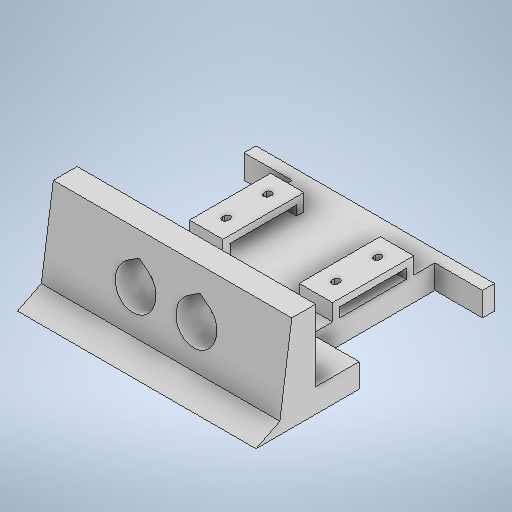
# Autodesk Inventor part: shell_01
Saved by Autodesk Inventor 2025.2 (Build 292293000, 293)
## iProperties
Created: 2025-11-21
Part Number: shell_01
Material: Generic
Document SubType Name: Modeling
Designer: Leo
Density: 1 g/cm^3
Appearance: Default
Author: Leo
Autodesk Inventor part; units mm, degrees
ref_plane "YZ Plane" through (0, 0, 0) normal (1, 0, 0) x (0, 1, 0)
ref_plane "XZ Plane" through (0, 0, 0) normal (0, 1, 0) x (-1, 0, 0)
ref_plane "XY Plane" through (0, 0, 0) normal (0, 0, 1) x (1, 0, 0)
sketch "Sketch3" plane through (0, 0, 0) normal (0, 1, 0) x (-1, 0, 0)
  line L0 (50, 50) -> (-50, 50)
  line L1 (-50, 50) -> (-50, -50)
  line L2 (-50, -50) -> (50, -50)
  line L3 (50, -50) -> (50, 50)
  line L4 (50, 50) -> (-50, -50) construction
  line L5 (-50, 50) -> (50, -50) construction
  line L6 (45, -45) -> (-45, 45) construction
  line L7 (-45, -45) -> (45, 45) construction
  point P0 (0, 0)
  dimension "d12" = 100
  dimension "d13" = 100
  constraints: 16 end point, 4 midpoint, 2 parallel, 1 horizontal, 1 perpendicular
  measures "d12" distance of L2.end L1.end
  measures "d13" distance of L0.end L1.end
extrude "Solid Mass" add sketch "Sketch3" along normal blind 40
sketch "Sketch6" plane through (50, 0, 50) normal (1, 0, 0) x (0, 0, -1)
  line L0 (0, 0) -> (100, 0) projected
  line L1 (0, 0) -> (10, 5)
  line L2 (10, 5) -> (15, 40)
  line L3 (0, 40) -> (100, 40) projected
  line L4 (0, 0) -> (0, 40)
  line L5 (100, 40) -> (25, 40)
  line L6 (25, 40) -> (25, 10)
  line L7 (25, 10) -> (100, 10)
  line L8 (100, 10) -> (100, 40)
  circle A0 centre (69.125, 22) radius 22.5
  line L9 (63.125, 17) -> (75.125, 17)
  line L10 (75.125, 17) -> (75.125, 27)
  line L11 (75.125, 27) -> (63.125, 27)
  line L12 (63.125, 27) -> (63.125, 17)
  line L13 (63.125, 17) -> (75.125, 27) construction
  line L14 (75.125, 17) -> (63.125, 27) construction
  line L15 (100, 0) -> (100, 40) projected
  line L16 (52.125, 10) -> (52.125, 17)
  line L17 (55.125, 10) -> (55.125, 14)
  line L18 (55.125, 14) -> (63.125, 14)
  line L19 (63.125, 14) -> (63.125, 10)
  line L20 (69.125, 22) -> (69.125, 0)
  line L21 (52.125, 17) -> (69.125, 17)
  line L22 (86.125, 10) -> (86.125, 17)
  line L23 (83.125, 10) -> (83.125, 14)
  line L24 (83.125, 14) -> (75.125, 14)
  line L25 (75.125, 14) -> (75.125, 10)
  line L26 (86.125, 17) -> (69.125, 17)
  point P0 (50, 0)
  point P1 (25, 40)
  point P2 (82.625, 40)
  point P3 (88.1579, 10)
  point P4 (64.408, 0)
  point P5 (50.0921, 10)
  point P6 (67.25, 14)
  point P7 (55.625, 40)
  point P8 (55.25, 14)
  point P9 (73.842, 0)
  point P10 (75.125, 10)
  point P11 (83.125, 10)
  point P12 (86.125, 10)
  point P13 (75.125, 17)
  dimension "d20" = 10
  dimension "d21" = 5
  dimension "d22" = 15
  dimension "d25" = 10
  dimension "d27" = 45
  dimension "d28" = 12
  dimension "d29" = 10
  dimension "d35" = 15
  dimension "d45" = 22
  dimension "d47" = 30.875
  dimension "d48" = 3
  dimension "d49" = 3
  dimension "d50" = 11
  constraints: 48 end point, 7 point on line, 6 symmetric about line, 5 perpendicular, 4 parallel, 4 vertical, 2 horizontal, 2 midpoint, 1 centre point, 1 collinear
  measures "d20" horizontal distance of L0.start L1.end
  measures "d21" vertical distance of L0.start L1.end
  measures "d22" horizontal distance of L0.start L2.end
  measures "d25" distance between parallel lines of L7 L0
  measures "d27" diameter of A0
  measures "d28" distance of L11.end L10.end
  measures "d29" distance of L10.end L9.end
  measures "d35" horizontal distance of L6.end L1.end
  measures "d45" distance from line of L0 L20.start
  measures "d47" distance of L0.end L20.end
  measures "d48" distance between parallel lines of L17 L16
  measures "d49" distance between parallel lines of L21 L18
  measures "d50" distance between parallel lines of L16 L19
extrude "Cut Ramp" cut sketch "Sketch6" against normal through all contours L4 L3 L2 L1 | A0 L3 L7 L22 L26 L10 L11 L12 L21 L16 | L7 L6 L3 A0 | L20 L9 L26 L22 L7 L23 L24 L25 | L7 L19 L18 L17 L16 L21 L9 L20 | A0 L3 L8 L7 | L7 L17 L18 L19 | L25 L24 L23 L7 | L9 L12 L11 L10
sketch "Sketch7" plane through (50, 10, 25) normal (0, 0, -1) x (-1, 0, 0)
  circle A0 centre (62.75, 11) radius 8.5
  line L0 (100, 0) -> (0, 0) projected
  line L1 (0, 30) -> (100, 30) projected
  line L2 (0, 0) -> (0, 30) projected
  line L3 (0, -10) -> (0, 0) projected
  line L4 (100, -10) -> (100, 0) projected
  line L5 (100, 30) -> (100, 0) projected
  line L6 (0, -10) -> (100, -10) projected
  line L7 (50, 30) -> (50, 0)
  circle A1 centre (37.25, 11) radius 8.5
  line L8 (58.2723, 18.225) -> (62.75, 21)
  line L9 (62.75, 21) -> (67.2277, 18.225)
  line L10 (41.7277, 18.225) -> (37.25, 21)
  line L11 (37.25, 21) -> (32.7723, 18.225)
  point P0 (50, -10)
  point P1 (32.7723, 18.225)
  point P2 (41.7277, 18.225)
  dimension "d30" = 17
  dimension "d31" = 11
  dimension "d32" = 25.5
  dimension "d46" = 10
  constraints: 10 end point, 4 symmetric about line, 2 centre point, 2 midpoint, 2 point on circle, 2 tangent, 1 vertical alignment, 1 other
  measures "d30" diameter of A0
  measures "d31" distance from line of L0 A0.centre
  measures "d32" diameter of A0.centre L7
  measures "d46" distance of A0.centre L8.end
extrude "Eyes" cut sketch "Sketch7" against normal through all contours A0 | A0 L8 L9 | A1 | A1 L11 L10
extrude "Motor Platform" add sketch "Sketch6" against normal up to surface (100 mm away) contours L20 L9 L26 L22 L7 L23 L24 L25 | L7 L19 L18 L17 L16 L21 L9 L20
sketch "Sketch9" plane through (-50, 0, -50) normal (-1, 0, 0) x (0, 0, 1)
  line L0 (5, 22) -> (5, 0)
  line L1 (56.75, 22) -> (56.75, 0)
  arc A0 (56.75, 22) -> (5, 22) centre (30.875, 22) ccw
  line L2 (5, 0) -> (56.75, 0)
  line L3 (0, 10) -> (13.875, 10) projected
  line L4 (24.875, 17) -> (24.875, 27) projected
  line L5 (24.875, 27) -> (36.875, 27) projected
  line L6 (36.875, 27) -> (36.875, 17) projected
  line L7 (13.875, 17) -> (47.875, 17) projected
  line L8 (13.875, 10) -> (0, 10) projected
  circle A1 centre (30.875, 22) radius 22.5 projected
  line L9 (0, 0) -> (100, 0) projected
  line L10 (0, 0) -> (0, 10) projected
  point P0 (50, 0)
  point P1 (5, 10)
  point P2 (26.158, 0)
  point P3 (11.8421, 10)
  point P4 (35.592, 0)
  dimension "d54" = 5
  dimension "d55" = 51.75
  dimension "d56" = 22
  constraints: 6 end point, 2 horizontal alignment, 2 point on circle, 1 centre point, 1 parallel, 1 point on line, 1 tangent, 1 vertical
  measures "d54" distance of L0.end L9.start
  measures "d55" distance of L0.start L1.start
  measures "d56" distance of L0.start L0.end
extrude "Cut right wheel" cut sketch "Sketch9" against normal blind 20 contours A0 L1 L2 A1 L3 L0 | L3 A1 L2 L0 | A1 L2 | L4 L5 L6 L7 picked at (31.5427, 32.8036)
extrude "Cut left wheel" cut sketch "Sketch9" along normal blind 20 from surface at -100 contours A0 L1 L2 A1 L3 L0 | L3 A1 L2 L0 | A1 L2 | L4 L5 L6 L7 picked at (31.5427, 32.8036)
sketch "Sketch8" plane through (50, 10, 25) normal (0, 1, 0) x (1, 0, 0)
  line L0 (-27, 35) -> (-27, 36) construction
  line L1 (-25.75, 35) -> (-25.75, 36)
  line L2 (-28.25, 36) -> (-28.25, 35)
  arc A0 (-28.25, 35) -> (-25.75, 35) centre (-27, 35) ccw
  arc A1 (-25.75, 36) -> (-28.25, 36) centre (-27, 36) ccw
  line L3 (-27, 52.5) -> (-27, 53.5) construction
  line L4 (-25.75, 52.5) -> (-25.75, 53.5)
  line L5 (-28.25, 53.5) -> (-28.25, 52.5)
  arc A2 (-28.25, 52.5) -> (-25.75, 52.5) centre (-27, 52.5) ccw
  arc A3 (-25.75, 53.5) -> (-28.25, 53.5) centre (-27, 53.5) ccw
  line L6 (-100, 0) -> (-100, 18.25) projected
  line L7 (0, 0) -> (-100, 0) projected
  line L8 (0, 75) -> (0, 70) projected
  line L9 (-100, 75) -> (0, 75) projected
  line L10 (-100, 75) -> (0, 75) projected
  line L11 (-50, 75) -> (-50, 0)
  line L12 (-73, 35) -> (-73, 36) construction
  line L13 (-74.25, 35) -> (-74.25, 36)
  line L14 (-71.75, 36) -> (-71.75, 35)
  arc A4 (-74.25, 35) -> (-71.75, 35) centre (-73, 35) ccw
  arc A5 (-71.75, 36) -> (-74.25, 36) centre (-73, 36) ccw
  line L15 (-73, 52.5) -> (-73, 53.5) construction
  line L16 (-74.25, 52.5) -> (-74.25, 53.5)
  line L17 (-71.75, 53.5) -> (-71.75, 52.5)
  arc A6 (-74.25, 52.5) -> (-71.75, 52.5) centre (-73, 52.5) ccw
  arc A7 (-71.75, 53.5) -> (-74.25, 53.5) centre (-73, 53.5) ccw
  line L18 (0, 0) -> (-100, 0) projected
  line L19 (-27, 0) -> (-27, 75) construction
  line L20 (-80, 18.25) -> (-100, 18.25) projected
  line L21 (0, 18.25) -> (0, 0) projected
  line L22 (0, 18.25) -> (-20, 18.25) projected
  line L23 (-20, 27.125) -> (-20, 18.25) projected
  line L24 (-20, 27.125) -> (-80, 27.125) projected
  line L25 (-80, 27.125) -> (-80, 18.25) projected
  line L26 (-100, 70) -> (-100, 75) projected
  line L27 (-100, 70) -> (-80, 70) projected
  line L28 (-80, 70) -> (-80, 61.125) projected
  line L29 (-80, 61.125) -> (-20, 61.125) projected
  line L30 (-20, 70) -> (-20, 61.125) projected
  line L31 (-20, 70) -> (0, 70) projected
  point P0 (-50, 25)
  point P1 (-27, 35.5)
  point P2 (-27, 53)
  point P3 (-73, 35.5)
  point P4 (-73, 53)
  point P5 (-50, 61.125)
  point P6 (-50, 27.125)
  dimension "d36" = 17.5
  dimension "d37" = 1.25
  dimension "d38" = 1
  dimension "d40" = 27
  dimension "d41" = 22
  constraints: 36 end point, 16 point on circle, 14 symmetric about line, 8 centre point, 8 tangent, 4 midpoint, 4 point on line, 2 parallel, 2 vertical, 1 collinear, 1 equal radius, 1 perpendicular, 4 other
  measures "d36" distance of point (-27, 53) point (-27, 35.5)
  measures "d37" radius of A0
  measures "d38" distance of L2.start L2.end
  measures "d40" distance between parallel lines of L8 L19
  measures "d41" distance from line of L9 point (-27, 53)
extrude "Cut Motor Bolt Holes" cut sketch "Sketch8" along normal blind 20 contours A0 L2 A1 L1 | A2 L5 A3 L4 | L13 A5 L14 A4 | L16 A7 L17 A6
sketch "Sketch10" plane through (-30, 10, -36.125) normal (0, 0, -1) x (-1, 0, 0)
  line L0 (-60, 0) -> (-60, 7) projected
  line L1 (-60, 7) -> (0, 7) projected
  line L2 (0, 0) -> (0, 7) projected
  line L3 (0, 0) -> (-60, 0) projected
  line L4 (-46, 7) -> (-14, 7)
  line L5 (-14, 7) -> (-14, 0)
  line L6 (-14, 0) -> (-46, 0)
  line L7 (-46, 0) -> (-46, 7)
  point P0 (-30, -10)
  point P1 (-46, 0)
  dimension "d61" = 14
  dimension "d62" = 14
  constraints: 8 end point, 2 parallel, 2 point on line, 1 horizontal, 1 perpendicular
  measures "d61" distance between parallel lines of L0 L7
  measures "d62" distance between parallel lines of L2 L5
extrude "Cut Centre" cut sketch "Sketch10" against normal up to surface (34 mm away) contours L7 L1 L5 L3
sketch "Sketch12" plane through (0, 0, 0) normal (0, -1, 0) x (1, 0, 0)
  line L0 (50, 25) -> (-50, 25) projected
  line L1 (-21.5, 18) -> (21.5, 18)
  line L2 (21.5, 18) -> (21.5, 6)
  line L3 (21.5, 6) -> (-21.5, 6)
  line L4 (-21.5, 6) -> (-21.5, 18)
  point P0 (0, 0)
  point P1 (0, 6)
  dimension "d72" = 43
  dimension "d73" = 12
  dimension "d74" = 7
  constraints: 8 end point, 2 parallel, 1 horizontal, 1 midpoint, 1 perpendicular, 1 vertical alignment
  measures "d72" distance of L1.start L1.end
  measures "d73" distance of L3.end L1.start
  measures "d74" distance between parallel lines of L0 L1
extrude "Extrusion13" cut sketch "Sketch12" against normal blind 10
sketch "Sketch13" plane through (50, 10, 25) normal (0, 0, -1) x (-1, 0, 0)
  line L0 (27.25, 21) -> (72.75, 21)
  line L1 (72.75, 21) -> (72.75, 1)
  line L2 (72.75, 1) -> (27.25, 1)
  line L3 (27.25, 1) -> (27.25, 21)
  arc A0 (58.2723, 18.225) -> (67.2277, 18.225) centre (62.75, 11) ccw projected
  circle A1 centre (62.75, 11) radius 10 construction
  arc A2 (32.7723, 18.225) -> (41.7277, 18.225) centre (37.25, 11) ccw projected
  circle A3 centre (37.25, 11) radius 10 construction
  line L4 (44, 5.5) -> (56, 5.5)
  line L5 (56, 5.5) -> (56, 1.5)
  line L6 (56, 1.5) -> (44, 1.5)
  line L7 (44, 1.5) -> (44, 5.5)
  circle A4 centre (54, 3.5) radius 2
  circle A5 centre (46, 3.5) radius 2
  line L8 (45, 20.5) -> (55, 20.5)
  line L9 (55, 20.5) -> (55, 17.5)
  line L10 (55, 17.5) -> (45, 17.5)
  line L11 (45, 17.5) -> (45, 20.5)
  point P0 (50, -10)
  point P1 (50, 5.5)
  point P2 (50, 1)
  point P3 (50, 20.5)
  point P4 (50, 21)
  point P5 (46, 1.5)
  point P6 (54, 1.5)
  point P7 (54, 5.5)
  point P8 (46, 5.5)
  dimension "d75" = 20
  dimension "d76" = 20
  dimension "d77" = 20
  dimension "d78" = 12
  dimension "d79" = 4
  dimension "d80" = 0.5
  dimension "d81" = 10
  dimension "d82" = 3
  dimension "d83" = 0.5
  constraints: 24 end point, 7 tangent, 6 parallel, 4 centre point, 4 midpoint, 3 horizontal, 3 perpendicular, 2 coincident, 2 vertical alignment
  measures "d75" distance of L0.end L1.end
  measures "d76" diameter of A1
  measures "d77" diameter of A3
  measures "d78" distance of L5.end L6.end
  measures "d79" distance of L6.end L4.start
  measures "d80" distance between parallel lines of L2 L6
  measures "d81" distance of L9.end L10.end
  measures "d82" distance of L10.end L8.start
  measures "d83" distance between parallel lines of L8 L0
extrude "Extrusion14" cut sketch "Sketch13" against normal blind 5 contours L4 A4 L6 A5 | A5 | A4 | L8 L9 L10 L11
sketch "Sketch16" plane through (-21.5, 0, 18) normal (1, 0, 0) x (0, 0, -1)
  line L0 (12, 0) -> (12, 10) projected
  line L1 (0, 0) -> (0, 10) projected
  line L2 (12, 0) -> (0, 0)
  line L3 (0, 0) -> (0, 4)
  line L4 (0, 4) -> (12, 4)
  line L5 (12, 4) -> (12, 0)
  point P0 (18, 0)
  dimension "d89" = 4
  constraints: 8 end point, 2 parallel, 1 horizontal, 1 perpendicular, 1 point on line
  measures "d89" distance of L2.end L3.end
extrude "Extrusion16" cut sketch "Sketch16" against normal blind 34
sketch "Sketch17" plane through (-50, 10, 25) normal (0, 1, 0) x (1, 0, 0)
  line L0 (20, 18.25) -> (0, 18.25) projected
  line L1 (0, 7) -> (71.5, 7) projected
  line L2 (0, 18.25) -> (10, 18.25)
  line L3 (10, 18.25) -> (10, 7)
  line L4 (10, 7) -> (0, 7)
  line L5 (0, 7) -> (0, 18.25)
  point P0 (50, 25)
  dimension "d92" = 10
  constraints: 8 end point, 2 parallel, 1 horizontal, 1 perpendicular, 1 point on line
  measures "d92" distance of L3.end L4.end
extrude "Extrusion17" cut sketch "Sketch17" against normal blind 34
sketch "Sketch18" plane through (-50, 10, 25) normal (0, 1, 0) x (1, 0, 0)
  line L0 (71.5, 7) -> (28.5, 7) projected
  line L1 (71.5, 19) -> (71.5, 7) projected
  line L2 (28.5, 19) -> (71.5, 19) projected
  line L3 (28.5, 7) -> (28.5, 19) projected
  line L4 (27.5, 6) -> (72.5, 6)
  line L5 (72.5, 6) -> (72.5, 20)
  line L6 (72.5, 20) -> (27.5, 20)
  line L7 (27.5, 20) -> (27.5, 6)
  point P0 (50, 25)
  dimension "d95" = 1
  constraints: 8 end point, 3 other
  measures "d95" distance between parallel lines of L0 L4
extrude "Extrusion18" add sketch "Sketch18" along normal blind 3
sketch "Sketch19" plane through (-50, 13, 25) normal (0, 1, 0) x (1, 0, 0)
  line L0 (28.5, 7) -> (28.5, 19) projected
  line L1 (71.5, 7) -> (28.5, 7)
  line L2 (28.5, 7) -> (28.5, 19)
  line L3 (28.5, 19) -> (71.5, 19)
  line L4 (71.5, 19) -> (71.5, 7)
  point P0 (50, 25)
  point P1 (28.5, 7)
  constraints: 8 end point, 2 parallel, 1 horizontal, 1 perpendicular
extrude "Extrusion19" add sketch "Sketch19" against normal blind 1.5
sketch "Sketch20" plane through (-30, 0, -50) normal (-1, 0, 0) x (0, 0, 1)
  line L0 (24.875, 14) -> (16.875, 14) projected
  line L1 (36.875, 10) -> (44.875, 10) projected
  line L2 (24.875, 14) -> (36.875, 14)
  line L3 (36.875, 14) -> (36.875, 10)
  line L4 (36.875, 10) -> (24.875, 10)
  line L5 (24.875, 10) -> (24.875, 14)
  point P0 (50, 0)
  constraints: 8 end point, 2 parallel, 1 horizontal, 1 perpendicular
extrude "Extrusion20" cut sketch "Sketch20" against normal blind 100
fillet "Fillet1" radius 3 1 edges at (0, 13, 19)
sketch "Sketch21" plane through (-50, 10, -50) normal (0, 1, 0) x (1, 0, 0)
  line L0 (59.9918, -13.8859) -> (42.201, -13.8859)
  line L1 (42.201, -13.8859) -> (42.201, -46.4739)
  line L2 (42.201, -46.4739) -> (59.9918, -46.4739)
  line L3 (59.9918, -46.4739) -> (59.9918, -13.8859)
  point P0 (50, -50)
  constraints: 8 end point, 2 parallel, 1 horizontal, 1 perpendicular
body "Solid2"
